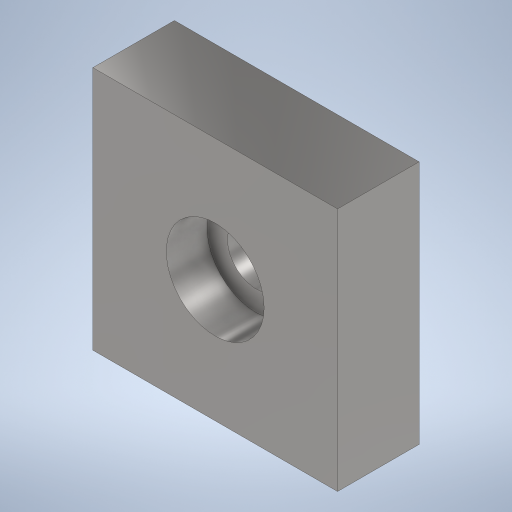
# Autodesk Inventor part: HCMUTE-CDT23-GOI_CHONG_QTAI
Saved by Autodesk Inventor 2023 (Build 270158000, 158)
## iProperties
Created: 2023-10-31
Part Number: HCMUTE-CDT23-GOI_CHONG_QTAI
Material: Stainless Steel
Document SubType Name: Modeling
Designer: havie
Density: 8 g/cm^3
Appearance: Semi-Polished
Mass: 66.1488 g
Surface Area: 32.2423 cm^2
Volume: 8.2686 cm^3
Author: havie
Autodesk Inventor part; units mm, degrees
ref_plane "YZ Plane" through (0, 0, 0) normal (1, 0, 0) x (0, 1, 0)
ref_plane "XZ Plane" through (0, 0, 0) normal (0, 1, 0) x (-1, 0, 0)
ref_plane "XY Plane" through (0, 0, 0) normal (0, 0, 1) x (1, 0, 0)
sketch "Sketch1" plane through (0, 0, 0) normal (0, 0, 1) x (1, 0, 0)
  line L0 (-15, 15) -> (15, 15)
  line L1 (15, 15) -> (15, -15)
  line L2 (15, -15) -> (-15, -15)
  line L3 (-15, -15) -> (-15, 15)
  line L4 (-15, 15) -> (15, -15) construction
  line L5 (15, 15) -> (-15, -15) construction
  point P0 (0, 0)
  dimension "d0" = 30
  dimension "d1" = 30
  constraints: 12 end point, 2 midpoint, 2 parallel, 1 horizontal, 1 perpendicular
  measures "d0" distance of L1.end L2.end
  measures "d1" distance of L0.end L1.end
extrude "Extrusion1" add sketch "Sketch1" along normal mid plane 10
sketch "Sketch2" plane through (0, 0, 5) normal (0, 0, 1) x (1, 0, 0)
  line L0 (-15, 15) -> (-15, -15) projected
  line L1 (15, 15) -> (-15, 15) projected
  point P0 (0, 0)
  point P1 (0, 0)
  point P2 (0, 15)
  dimension "d13" = 15
  dimension "d15" = 15
  constraints: 1 midpoint
  measures "d13" distance from line of L0 point (0, 0)
  measures "d15" distance from line of L1 point (0, 0)
hole "Hole1" at (0, 0, 5) direction (0, 0, -1) diameter 7 end through all counterbore diameter 12 counterbore depth 5
body "Solid1"
